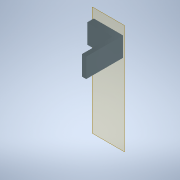
# Autodesk Inventor part: silla
Saved by Autodesk Inventor 2021 (Build 250183000, 183)
## iProperties
Created: 2021-03-18
Part Number: silla
Material: Lead
Document SubType Name: Modeling
Designer: andre
Density: 11.34 g/cm^3
Appearance: Lead
Author: andre
Autodesk Inventor part; units mm, degrees
ref_plane "YZ Plane" through (0, 0, 0) normal (1, 0, 0) x (0, 1, 0)
ref_plane "XZ Plane" through (0, 0, 0) normal (0, 1, 0) x (-1, 0, 0)
ref_plane "XY Plane" through (0, 0, 0) normal (0, 0, 1) x (1, 0, 0)
ref_plane "Work Plane1" through (0, 0, 0) normal (0, 0, 1) x (1, 0, 0)
sketch "Sketch1" plane through (0, 0, 0) normal (0, 0, 1) x (1, 0, 0)
  line L0 (-337.5, 1114) -> (337.5, 1114)
  line L1 (-337.5, 1114) -> (337.5, 1114)
  line L2 (337.5, 584) -> (-337.5, 584)
  line L3 (337.5, 584) -> (-337.5, 584)
  line L4 (-337.5, 584) -> (-337.5, 1114)
  line L5 (-337.5, 1114) -> (337.5, 1114)
  line L6 (337.5, 1114) -> (337.5, 584)
  point P0 (0, 0)
  constraints: 14 end point, 4 horizontal, 2 parallel, 1 perpendicular, 4 other
extrude "Extrusion1" add sketch "Sketch1" along normal blind 150
sketch "Sketch2" plane through (0, 0, 150) normal (0, 0, 1) x (1, 0, 0)
  line L0 (-337.5, 584) -> (337.5, 584) projected
  line L1 (337.5, 1114) -> (-337.5, 1114) projected
  line L2 (337.5, 584) -> (187.5, 584)
  line L3 (187.5, 584) -> (187.5, 1114)
  line L4 (187.5, 1114) -> (337.5, 1114)
  line L5 (337.5, 1114) -> (337.5, 584)
  point P0 (0, 0)
  point P1 (187.5, 584)
  dimension "d6" = 150
  constraints: 8 end point, 2 parallel, 1 horizontal, 1 perpendicular, 1 point on line
  measures "d6" distance of L3.end L4.end
extrude "Extrusion2" add sketch "Sketch2" along normal blind 700
body "Solid1"
